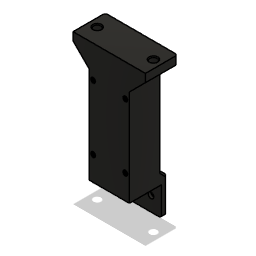
Base support (Autodesk Fusion 360 design; units mm, degrees)
Autodesk Fusion 360 part; units mm, degrees
sketch "Sketch1" plane through (0, 0, 0) normal (0, 0, 1) x (1, 0, 0)
  line L0 (0, 0) -> (25, 0)
  line L1 (25, 0) -> (25, 70)
  line L2 (25, 70) -> (0, 70) construction
  line L3 (0, 70) -> (0, 0)
  line L4 (25, 70) -> (35, 70)
  line L5 (35, 70) -> (35, 75)
  line L6 (35, 75) -> (-10, 75)
  line L7 (0, 70) -> (-10, 70)
  line L8 (-10, 70) -> (-10, 75)
  dimension "d1" = 25
  dimension "d2" = 70
  dimension "d3" = 10
  dimension "d4" = 5
  dimension "d5" = 10
  constraint horizontal L0
  constraint vertical L1
  constraint horizontal L2
  constraint vertical L3
  constraint coincident L0.start L3.end
  constraint perpendicular L1 L4
  constraint perpendicular L4 L5
  constraint perpendicular L5 L6
  constraint perpendicular L3 L7
  constraint perpendicular L7 L8
  constraint coincident L6.end L8.end
  measures "d1" distance of L0.start L0.end
  measures "d2" distance of L0.start L2.end
  measures "d3" distance of L1.end L4.end
  measures "d4" distance of L4.end L5.end
  measures "d5" distance of L2.end L7.end
extrude "Extrude1" add sketch "Sketch1" along normal blind 20
chamfer "Chamfer1" distance 10 angle 45 2 edges at (0, 70, 10) (25, 70, 10)
sketch "Sketch2" plane through (0, 75, 0) normal (0, 1, 0) x (-1, 0, 0)
  line L0 (-35, 0) -> (10, 0)
  line L1 (10, 0) -> (10, 20)
  line L2 (10, 20) -> (-35, 20)
  line L3 (-35, 20) -> (-35, 0)
  line L4 (10, 10) -> (-35, 10) construction
  circle A0 centre (5, 10) radius 2.25
  circle A1 centre (-30, 10) radius 2.25
  line L5 (-12.5, 0) -> (-12.5, 20) construction
  dimension "d9" = 4.5
  dimension "d10" = 4.5
  dimension "d11" = 5
  constraint midpoint L1 L4.start
  constraint midpoint L3 L4.end
  constraint coincident L4 A0.centre
  constraint coincident L4 A1.centre
  constraint midpoint L0 L5.start
  constraint midpoint L2 L5.end
  constraint symmetric A0 A1 L5
  measures "d9" diameter of A0
  measures "d10" diameter of A1
  measures "d11" distance of L3 A1.centre
extrude "Extrude2" cut sketch "Sketch2" against normal blind 25 contours A0 | A1
sketch "Sketch3" plane through (0, 75, 0) normal (0, 1, 0) x (-1, 0, 0)
  circle A0 centre (-30, 10) radius 2.25
  circle A1 centre (5, 10) radius 2.25
  line L0 (-35, 0) -> (10, 0)
  line L1 (10, 0) -> (10, 20)
  line L2 (10, 20) -> (-35, 20)
  line L3 (-35, 20) -> (-35, 0)
  circle A2 centre (5, 10) radius 4
  circle A3 centre (-30, 10) radius 4
  dimension "d14" = 8
  dimension "d15" = 8
  constraint concentric A1 A2
  constraint concentric A0 A3
  measures "d14" diameter of A2
  measures "d15" diameter of A3
extrude "Extrude3" cut sketch "Sketch3" against normal blind 21 from surface at -5.75 contours A2 | A3
sketch "Sketch4" plane through (25, 0, 0) normal (1, 0, 0) x (0, 0, -1)
  line L0 (-20, 60) -> (-20, 0)
  line L1 (-20, 0) -> (0, 0)
  line L2 (0, 0) -> (0, 60)
  line L3 (0, 7) -> (3.5, 3.5)
  line L4 (3.5, 3.5) -> (3.5, -18)
  line L5 (3.5, -18) -> (0, -18)
  line L6 (0, -18) -> (0, 0)
  line L7 (0, 60) -> (-20, 60)
  dimension "d19" = 18
  dimension "d20" = 3.5
  dimension "d21" = 3.5
  dimension "d22" = 45
  constraint coincident L2 L3.start
  constraint parallel L2 L4
  constraint perpendicular L2 L5
  constraint coincident L1.end L2.start
  constraint perpendicular L1 L6
  measures "d19" distance of L5.end L1.end
  measures "d20" distance of L4 L6
  measures "d21" vertical distance of L3.end L1.end
  measures "d22" angle of L3 L4
extrude "Extrude4" add sketch "Sketch4" against normal blind 25 contours L2 L3 L4 L5 L6
chamfer "Chamfer2" distance 1 angle 45 13 edges at (35, 72.5, 0) (30, 65, 0) (25, 33.5, 0) (25, 5.25, -1.75) (25, -7.25, -3.5) (0, -7.25, -3.5) (0, 5.25, -1.75) (0, 33.5, 0) (-5, 65, 0) (-10, 72.5, 0) (12.5, -18, -3.5) (25, -18, -1.75) (0, -18, -1.75)
sketch "Sketch5" plane through (0, 0, 0) normal (0, 0, 1) x (1, 0, 0)
  line L0 (24, -18) -> (25, -17)
  line L1 (25, -17) -> (25, 0)
  line L2 (25, 0) -> (0, 0)
  line L3 (0, 0) -> (0, -17)
  line L4 (0, -17) -> (1, -18)
  line L5 (1, -18) -> (24, -18)
  line L6 (0, -9) -> (25, -9) construction
  circle A0 centre (6.5, -9) radius 1.75
  circle A1 centre (18.5, -9) radius 1.75
  dimension "d26" = 3.5
  dimension "d27" = 3.5
  dimension "d28" = 6.5
  dimension "d29" = 6.5
  dimension "d42" = 9
  constraint coincident L6 A0.centre
  constraint coincident L6 A1.centre
  measures "d26" diameter of A0
  measures "d27" diameter of A1
  measures "d28" distance of L1 A1.centre
  measures "d29" distance of L3 A0.centre
  measures "d42" distance of L5 L6
extrude "Extrude5" cut sketch "Sketch5" against normal blind 3.5 contours A0 | A1
chamfer "Chamfer3" distance 1.75 angle 45 2 edges at (4.8684, -9.6328, -3.5) (16.8684, -9.6328, -3.5)
sketch "Sketch6" plane through (0, 0, 20) normal (0, 0, 1) x (1, 0, 0)
  line L0 (0, 60) -> (0, 0)
  line L1 (0, 0) -> (25, 0)
  line L2 (25, 0) -> (25, 60)
  line L3 (35, 70) -> (35, 75)
  line L4 (35, 75) -> (-10, 75)
  line L5 (-10, 75) -> (-10, 70)
  line L6 (12.5, 75) -> (12.5, 0) construction
  line L7 (22.5, 15) -> (2.5, 15) construction
  line L8 (2.5, 15) -> (2.5, 55) construction
  line L9 (2.5, 55) -> (22.5, 55) construction
  line L10 (22.5, 55) -> (22.5, 15) construction
  line L11 (22.5, 15) -> (2.5, 55) construction
  line L12 (2.5, 15) -> (22.5, 55) construction
  circle A0 centre (22.5, 55) radius 1.5
  circle A1 centre (2.5, 55) radius 1.5
  circle A2 centre (2.5, 15) radius 1.5
  circle A3 centre (22.5, 15) radius 1.5
  line L13 (25, 60) -> (35, 70)
  line L14 (-10, 70) -> (0, 60)
  point P0 (12.5, 35)
  dimension "d33" = 20
  dimension "d34" = 40
  dimension "d35" = 15
  dimension "d36" = 3
  dimension "d37" = 3
  dimension "d38" = 3
  dimension "d39" = 3
  constraint midpoint L4 L6.start
  constraint midpoint L1 L6.end
  constraint horizontal L7
  constraint perpendicular L7 L8
  constraint parallel L7 L9
  constraint parallel L8 L10
  constraint coincident L11 P0
  constraint coincident L12 P0
  constraint coincident L6 P0
  constraint coincident L9.end L10.start
  constraint coincident L8.end L9.start
  constraint coincident L7.end L8.start
  constraint coincident L7.start L10.end
  measures "d33" distance of L8.end L9.end
  measures "d34" distance of L7.end L8.end
  measures "d35" distance of L1 L7
  measures "d36" diameter of A0
  measures "d37" diameter of A1
  measures "d38" diameter of A2
  measures "d39" diameter of A3
extrude "Extrude6" cut sketch "Sketch6" against normal blind 10 contours A0 | A1 | A2 | A3
thread "Thread1" "ISO Metric profile 3.0 M3x0.5 6H" major diameter 3.086 minor diameter 2.529 pitch 0.5 angle 60 modelled right hand crest width 0.1368 on face at (1.0905, 54.487, 13.3333) crest through (3.7645, 55, 19.875) on face at (21.2201, 54.2178, 13.3333) crest through (23.7645, 55, 19.875) on face at (23.9981, 14.9252, 13.3333) crest through (23.7645, 15, 19.875) on face at (3.9981, 14.9252, 13.3333) crest through (3.7645, 15, 19.875)
chamfer "Chamfer4" distance 0.5 angle 45 2 edges at (-2.9023, 75, 10.8136) (32.0977, 75, 10.8136)
